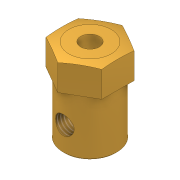
# Autodesk Inventor part: Coupler
Saved by Autodesk Inventor 2020 (Build 240168000, 168)
## iProperties
Created: 2022-03-01
Part Number: Coupler
Material: Generic
Document SubType Name: Modeling
Designer: ferrerx
Density: 1 g/cm^3
Appearance: Brass - Satin
Author: ferrerx
Autodesk Inventor part; units mm, degrees
ref_plane "YZ Plane" through (0, 0, 0) normal (1, 0, 0) x (0, 1, 0)
ref_plane "XZ Plane" through (0, 0, 0) normal (0, 1, 0) x (-1, 0, 0)
ref_plane "XY Plane" through (0, 0, 0) normal (0, 0, 1) x (1, 0, 0)
sketch "Sketch1" plane through (0, 0, 0) normal (0, 1, 0) x (-1, 0, 0)
  circle A0 centre (0, 0) radius 5.75
  circle A1 centre (0, 0) radius 2
  dimension "d0" = 4
  dimension "d1" = 11.5
  constraints: 2 centre point, 2 coincident
  measures "d0" diameter of A1
  measures "d1" diameter of A0
extrude "Extrusion1" add sketch "Sketch1" along normal blind 12
sketch "Sketch2" plane through (0, 12, 0) normal (0, 1, 0) x (1, 0, 0)
  circle A0 centre (0, 0) radius 2
  line L0 (0, 6.9282) -> (6, 3.4641)
  line L1 (6, 3.4641) -> (6, -3.4641)
  line L2 (6, -3.4641) -> (0, -6.9282)
  line L3 (0, -6.9282) -> (-6, -3.4641)
  line L4 (-6, -3.4641) -> (-6, 3.4641)
  line L5 (-6, 3.4641) -> (0, 6.9282)
  dimension "d4" = 12
  constraints: 12 end point, 2 coincident, 1 centre point, 13 other
  measures "d4" distance between parallel lines of L4 L1
extrude "Extrusion2" add sketch "Sketch2" along normal blind 6
chamfer "Chamfer1" distance 0.3 angle 45 1 edges at (5.75, 0, 0)
sketch "Sketch3" plane through (0, 0, 0) normal (1, 0, 0) x (0, 1, 0)
  line L0 (16.8879, 9.0352) -> (19.8879, 9.0352)
  line L1 (18, 2) -> (18, -2) projected
  line L2 (18, 3.4641) -> (18, 6.9282) projected
  line L3 (-31.6303, 0) -> (26.5625, 0) projected
  line L4 (19.8879, 9.0352) -> (19.8879, 0)
  line L5 (19.8879, 0) -> (18, 0)
  arc A0 (18, 0) -> (16.8879, 9.0352) centre (-0.7575, 2.2772) ccw
  point P0 (0, 0)
  dimension "d10" = 9.0352
  dimension "d11" = 3
  constraints: 6 end point, 2 midpoint, 2 point on circle, 1 centre point, 1 horizontal, 1 perpendicular
  measures "d10" distance from line of L5.end L0
  measures "d11" distance of L0.start L0.end
revolve "Revolution1" cut sketch "Sketch3" angle 360 about axis through (0, 0, 0) along (0, 1, 0)
sketch "Sketch4" plane through (0, 0, 0) normal (0, 0, 1) x (1, 0, 0)
  line L0 (0, 0) -> (0, 5.3666) construction
  circle A0 centre (0, 5.3666) radius 2
  dimension "d13" = 4
  constraints: 2 end point, 1 centre point, 1 coincident
  measures "d13" diameter of A0
extrude "Extrusion3" cut sketch "Sketch4" against normal mid plane 30
thread "Thread1" size "M4x0.7" class "6H" standard "ANSI Metric M Profile" length 180
thread "Thread2" size "M4x0.7" class "6H" standard "ANSI Metric M Profile" length 180
body "Solid1"
